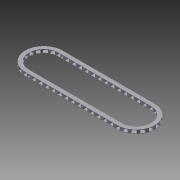
# Autodesk Inventor part: chain
Saved by Autodesk Inventor 2011 (Build 150239000, 239)
## iProperties
Created: 2010-04-19
Part Number: chain
Document SubType Name: Modeling
Designer: lucio
Density: 2.71 g/cm^3
Material: Aluminum-6061
Author: lucio
Autodesk Inventor part; units mm, degrees
ref_plane "YZ Plane" through (0, 0, 0) normal (1, 0, 0) x (0, 1, 0)
ref_plane "XZ Plane" through (0, 0, 0) normal (0, 1, 0) x (-1, 0, 0)
ref_plane "XY Plane" through (0, 0, 0) normal (0, 0, 1) x (1, 0, 0)
sketch "Sketch1" plane through (0, 0, 0) normal (0, 0, 1) x (1, 0, 0)
  line L0 (25, 0) -> (150, 0)
  line L1 (175, 25) -> (175, 25)
  line L2 (150, 50) -> (25, 50)
  line L3 (0, 25) -> (0, 25)
  arc A0 (25, 50) -> (0, 25) centre (25, 25) ccw
  arc A1 (175, 25) -> (150, 50) centre (150, 25) ccw
  arc A2 (150, 0) -> (175, 25) centre (150, 25) ccw
  arc A3 (0, 25) -> (25, 0) centre (25, 25) ccw
  line L4 (25, 45) -> (150, 45)
  line L5 (170, 25) -> (170, 25)
  line L6 (150, 5) -> (25, 5)
  line L7 (5, 25) -> (5, 25)
  arc A4 (25, 45) -> (5, 25) centre (25, 25) ccw
  arc A5 (5, 25) -> (25, 5) centre (25, 25) ccw
  arc A6 (150, 5) -> (170, 25) centre (150, 25) ccw
  arc A7 (170, 25) -> (150, 45) centre (150, 25) ccw
  line L8 (22.5, 25) -> (27.5, 25)
  line L9 (27.5, 25) -> (27.5, 50)
  line L10 (27.5, 50) -> (22.5, 50)
  line L11 (22.5, 50) -> (22.5, 25)
  line L12 (22.6508, 24.1449) -> (27.3492, 25.8551)
  line L13 (27.3492, 25.8551) -> (18.7987, 49.3474)
  line L14 (18.7987, 49.3474) -> (14.1003, 47.6373)
  line L15 (14.1003, 47.6373) -> (22.6508, 24.1449)
  line L16 (23.0849, 23.393) -> (26.9151, 26.607)
  line L17 (26.9151, 26.607) -> (10.8454, 45.7581)
  line L18 (10.8454, 45.7581) -> (7.0152, 42.5441)
  line L19 (7.0152, 42.5441) -> (23.0849, 23.393)
  line L20 (23.75, 22.8349) -> (26.25, 27.1651)
  line L21 (26.25, 27.1651) -> (4.5994, 39.6651)
  line L22 (4.5994, 39.6651) -> (2.0994, 35.3349)
  line L23 (2.0994, 35.3349) -> (23.75, 22.8349)
  line L24 (24.5659, 22.538) -> (25.4341, 27.462)
  line L25 (25.4341, 27.462) -> (0.8139, 31.8032)
  line L26 (0.8139, 31.8032) -> (-0.0543, 26.8792)
  line L27 (-0.0543, 26.8792) -> (24.5659, 22.538)
  line L28 (25.4341, 22.538) -> (24.5659, 27.462)
  line L29 (24.5659, 27.462) -> (-0.0543, 23.1208)
  line L30 (-0.0543, 23.1208) -> (0.8139, 18.1968)
  line L31 (0.8139, 18.1968) -> (25.4341, 22.538)
  line L32 (26.25, 22.8349) -> (23.75, 27.1651)
  line L33 (23.75, 27.1651) -> (2.0994, 14.6651)
  line L34 (2.0994, 14.6651) -> (4.5994, 10.3349)
  line L35 (4.5994, 10.3349) -> (26.25, 22.8349)
  line L36 (26.9151, 23.393) -> (23.0849, 26.607)
  line L37 (23.0849, 26.607) -> (7.0152, 7.4559)
  line L38 (7.0152, 7.4559) -> (10.8454, 4.2419)
  line L39 (10.8454, 4.2419) -> (26.9151, 23.393)
  line L40 (27.3492, 24.1449) -> (22.6508, 25.8551)
  line L41 (22.6508, 25.8551) -> (14.1003, 2.3627)
  line L42 (14.1003, 2.3627) -> (18.7987, 0.6526)
  line L43 (18.7987, 0.6526) -> (27.3492, 24.1449)
  line L44 (27.5, 25) -> (22.5, 25)
  line L45 (22.5, 25) -> (22.5, 0)
  line L46 (22.5, 0) -> (27.5, 0)
  line L47 (27.5, 0) -> (27.5, 25)
  line L48 (147.5, 24.9667) -> (152.5, 24.9667)
  line L49 (152.5, 24.9667) -> (152.5, 51.0386)
  line L50 (152.0822, 51.0326) -> (147.5, 50.9667)
  line L51 (147.5, 50.9667) -> (147.5, 24.9667)
  line L52 (147.6394, 25.8238) -> (152.3379, 24.1137)
  line L53 (152.3379, 24.1137) -> (161.255, 48.6133)
  line L54 (161.255, 48.6133) -> (156.5319, 50.2558)
  line L55 (156.5319, 50.2558) -> (147.6394, 25.8238)
  line L56 (148.0635, 26.5815) -> (151.8937, 23.3676)
  line L57 (151.8937, 23.3676) -> (168.6524, 43.3398)
  line L58 (168.6524, 43.3398) -> (164.776, 46.4986)
  line L59 (164.776, 46.4986) -> (148.0635, 26.5815)
  line L60 (148.7212, 27.1484) -> (151.2212, 22.8183)
  line L61 (151.2212, 22.8183) -> (173.8001, 35.8543)
  line L62 (173.8001, 35.8543) -> (171.2379, 40.1484)
  line L63 (171.2379, 40.1484) -> (148.7212, 27.1484)
  line L64 (149.5331, 27.4562) -> (150.4014, 22.5322)
  line L65 (150.4014, 22.5322) -> (176.0772, 27.0595)
  line L66 (176.0772, 27.0595) -> (175.1381, 31.9711)
  line L67 (175.1381, 31.9711) -> (149.5331, 27.4562)
  line L68 (150.4014, 27.4678) -> (149.5331, 22.5438)
  line L69 (149.5331, 22.5438) -> (175.2089, 18.0164)
  line L70 (175.2089, 18.0164) -> (176.0064, 22.9529)
  line L71 (176.0064, 22.9529) -> (150.4014, 27.4678)
  line L72 (151.2212, 27.1817) -> (148.7212, 22.8516)
  line L73 (148.7212, 22.8516) -> (171.3001, 9.8156)
  line L74 (171.3001, 9.8156) -> (173.7379, 14.1817)
  line L75 (173.7379, 14.1817) -> (151.2212, 27.1817)
  line L76 (151.8937, 26.6324) -> (148.0635, 23.4185)
  line L77 (148.0635, 23.4185) -> (164.8222, 3.4463)
  line L78 (164.8222, 3.4463) -> (168.6062, 6.7153)
  line L79 (168.6062, 6.7153) -> (151.8937, 26.6324)
  line L80 (152.3379, 25.8863) -> (147.6394, 24.1762)
  line L81 (147.6394, 24.1762) -> (156.5565, -0.3234)
  line L82 (156.5565, -0.3234) -> (161.2304, 1.4543)
  line L83 (161.2304, 1.4543) -> (152.3379, 25.8863)
  line L84 (152.5, 25.0333) -> (147.5, 25.0333)
  line L85 (147.5, 25.0333) -> (147.5, -1.0386)
  line L86 (147.5, -1.0386) -> (152.5, -0.9667)
  line L87 (152.5, -0.9667) -> (152.5, 25.0333)
  line L88 (143.785, 50) -> (138.785, 50)
  line L89 (138.785, 50) -> (138.785, -0.7152)
  line L90 (138.785, -0.7152) -> (143.785, -0.7152)
  line L91 (143.785, -0.7152) -> (143.785, 50)
  line L92 (135.07, 50) -> (130.07, 50)
  line L93 (130.07, 50) -> (130.07, 0)
  line L94 (130.07, 0) -> (135.07, 0)
  line L95 (135.07, 0) -> (135.07, 50)
  line L96 (126.355, 0) -> (121.355, 0)
  line L97 (121.355, 0) -> (121.355, 50)
  line L98 (121.355, 50) -> (126.355, 50)
  line L99 (126.355, 50) -> (126.355, 0)
  line L100 (117.64, 50) -> (112.64, 50)
  line L101 (112.64, 50) -> (112.64, 0)
  line L102 (112.64, 0) -> (117.64, 0)
  line L103 (117.64, 0) -> (117.64, 50)
  line L104 (108.925, 50) -> (103.925, 50)
  line L105 (103.925, 50) -> (103.925, 0)
  line L106 (103.925, 0) -> (108.925, 0)
  line L107 (108.925, 0) -> (108.925, 50)
  line L108 (100.21, 50) -> (95.21, 50)
  line L109 (95.21, 50) -> (95.21, 0)
  line L110 (95.21, 0) -> (100.21, 0)
  line L111 (100.21, 0) -> (100.21, 50)
  line L112 (91.495, 50) -> (86.495, 50)
  line L113 (86.495, 50) -> (86.495, 0)
  line L114 (86.495, 0) -> (91.495, 0)
  line L115 (91.495, 0) -> (91.495, 50)
  line L116 (82.78, 50) -> (77.78, 50)
  line L117 (77.78, 50) -> (77.78, 0)
  line L118 (77.78, 0) -> (82.78, 0)
  line L119 (82.78, 0) -> (82.78, 50)
  line L120 (74.065, 50) -> (69.065, 50)
  line L121 (69.065, 50) -> (69.065, 0)
  line L122 (69.065, 0) -> (74.065, 0)
  line L123 (74.065, 0) -> (74.065, 50)
  line L124 (65.35, 50) -> (60.35, 50)
  line L125 (60.35, 50) -> (60.35, 0)
  line L126 (60.35, 0) -> (65.35, 0)
  line L127 (65.35, 0) -> (65.35, 50)
  line L128 (56.635, 50) -> (51.635, 50)
  line L129 (51.635, 50) -> (51.635, 0)
  line L130 (51.635, 0) -> (56.635, 0)
  line L131 (56.635, 0) -> (56.635, 50)
  line L132 (47.92, 50) -> (42.92, 50)
  line L133 (42.92, 50) -> (42.92, 0)
  line L134 (42.92, 0) -> (47.92, 0)
  line L135 (47.92, 0) -> (47.92, 50)
  line L136 (39.205, 50) -> (34.205, 50)
  line L137 (34.205, 50) -> (34.205, 0)
  line L138 (34.205, 0) -> (39.205, 0)
  line L139 (39.205, 0) -> (39.205, 50)
  line L140 (30.49, 50) -> (27.6882, 50)
  line L141 (27.6882, 50) -> (27.6882, 0)
  line L142 (27.6882, 0) -> (30.49, 0)
  line L143 (30.49, 0) -> (30.49, 50)
  line L144 (152.0822, 51.0326) -> (147.5, 51.0326)
  line L145 (147.5, 51.0326) -> (147.5, 25.0333)
  line L146 (147.5, 25.0333) -> (152.0822, 25.0333)
  line L147 (152.0822, 25.0333) -> (152.0822, 51.0326)
  point P0 (0, 0)
  point P1 (175, 50)
  point P2 (175, 0)
  point P3 (0, 50)
  point P4 (170, 5)
  point P5 (170, 45)
  point P6 (5, 5)
  point P7 (16.4495, 48.4923)
  point P8 (18.1596, 43.7939)
  point P9 (8.9303, 44.1511)
  point P10 (12.1442, 40.3209)
  point P11 (3.3494, 37.5)
  point P12 (7.6795, 35)
  point P13 (0.3798, 29.3412)
  point P14 (5.3038, 28.473)
  point P15 (0.3798, 20.6588)
  point P16 (5.3038, 21.527)
  point P17 (3.3494, 12.5)
  point P18 (7.6795, 15)
  point P19 (8.9303, 5.8489)
  point P20 (12.1442, 9.6791)
  point P21 (16.4495, 1.5077)
  point P22 (18.1596, 6.2061)
  point P23 (25, 0)
  point P24 (25, 5)
  point P25 (158.5505, 48.4923)
  point P26 (156.8404, 43.7939)
  point P27 (166.0697, 44.1511)
  point P28 (162.8558, 40.3209)
  point P29 (171.6506, 37.5)
  point P30 (167.3205, 35)
  point P31 (174.6202, 29.3412)
  point P32 (169.6962, 28.473)
  point P33 (174.6202, 20.6588)
  point P34 (169.6962, 21.527)
  point P35 (171.6506, 12.5)
  point P36 (167.3205, 15)
  point P37 (166.0697, 5.8489)
  point P38 (162.8558, 9.6791)
  point P39 (158.5505, 1.5077)
  point P40 (156.8404, 6.2061)
  point P41 (150, 5)
  dimension "d0" = 175
  dimension "d1" = 50
  dimension "d2" = 25
  dimension "d3" = 165
  dimension "d4" = 40
  dimension "d6" = 20
  dimension "d11" = 2.5
  dimension "d12" = 5
  dimension "d15" = 180
  dimension "d19" = 2.5
  dimension "d20" = 5
  dimension "d23" = 180
  dimension "d27" = 5
  dimension "d28" = 3.715
  dimension "d29" = 3.715
  dimension "d30" = 3.715
  dimension "d31" = 5
  dimension "d32" = 5
  dimension "d33" = 3.715
  dimension "d34" = 5
  dimension "d35" = 3.715
  dimension "d36" = 5
  dimension "d37" = 3.715
  dimension "d38" = 5
  dimension "d39" = 3.715
  dimension "d40" = 5
  dimension "d41" = 3.715
  dimension "d42" = 5
  dimension "d43" = 3.715
  dimension "d44" = 5
  dimension "d45" = 3.715
  dimension "d46" = 5
  dimension "d47" = 3.715
  dimension "d48" = 5
  dimension "d49" = 3.715
  dimension "d50" = 5
  dimension "d51" = 3.715
  dimension "d52" = 5
  dimension "d53" = 2.8018
  dimension "d54" = 3.715
  dimension "d59" = 26
  dimension "d60" = 26
  constraints: 292 end point, 35 parallel, 18 horizontal, 18 perpendicular, 16 point on circle, 12 coincident, 12 tangent, 10 point on line, 8 centre point, 6 equal radius, 1 vertical, 294 other
  measures "d0" distance of point (0, 50) point (175, 50)
  measures "d1" distance of point (175, 50) point (175, 0)
  measures "d2" radius of A0
  measures "d3" distance of point (170, 5) point (5, 5)
  measures "d4" distance of point (170, 45) point (170, 5)
  measures "d6" radius of A4
  measures "d11" distance from line of A0.centre L11
  measures "d12" distance between parallel lines of L11 L9
  measures "d19" distance from line of L51 A1.centre
  measures "d20" distance between parallel lines of L49 L51
  measures "d27" distance between parallel lines of L91 L89
  measures "d28" distance between parallel lines of L51 L91
  measures "d29" distance between parallel lines of L99 L93
  measures "d30" distance between parallel lines of L95 L89
  measures "d31" distance between parallel lines of L93 L95
  measures "d32" distance between parallel lines of L97 L99
  measures "d33" distance between parallel lines of L103 L97
  measures "d34" distance between parallel lines of L101 L103
  measures "d35" distance between parallel lines of L107 L101
  measures "d36" distance between parallel lines of L105 L107
  measures "d37" distance between parallel lines of L111 L105
  measures "d38" distance between parallel lines of L109 L111
  measures "d39" distance between parallel lines of L109 L115
  measures "d40" distance between parallel lines of L113 L115
  measures "d41" distance between parallel lines of L119 L113
  measures "d42" distance between parallel lines of L117 L119
  measures "d43" distance between parallel lines of L123 L117
  measures "d44" distance between parallel lines of L121 L123
  measures "d45" distance between parallel lines of L127 L121
  measures "d46" distance between parallel lines of L125 L127
  measures "d47" distance between parallel lines of L131 L125
  measures "d48" distance between parallel lines of L129 L131
  measures "d49" distance between parallel lines of L135 L129
  measures "d50" distance between parallel lines of L133 L135
  measures "d51" distance between parallel lines of L133 L139
  measures "d52" distance between parallel lines of L137 L139
  measures "d53" distance between parallel lines of L141 L143
  measures "d54" distance between parallel lines of L143 L137
  measures "d59" distance of L50.end L48.start
  measures "d60" distance from line of A1.centre L50
extrude "Extrusion1" add sketch "Sketch1" along normal mid plane 5 contours A3 L45 A5 L6 L47 L0 | L47 L6 L141 L0 | A3 L43 A5 L45 | L141 L6 L143 L0 | A3 L41 A5 L43 | L143 L6 L137 L0 | L137 L6 L139 L0 | L141 L2 L143 L4 | L4 L9 L2 L141 | L4 A4 L11 A0 L2 L9 | A3 L39 A5 L41 | L139 L6 L133 L0 | L143 L2 L137 L4 | A3 L37 A5 L39 | L133 L6 L135 L0 | L137 L2 L139 L4 | A4 L13 A0 L11 | L37 A3 L35 A5 | L135 L6 L129 L0 | L139 L2 L133 L4 | A4 L15 A0 L13 | L35 A3 L33 A5 | L129 L6 L131 L0 | L133 L2 L135 L4 | A4 L17 A0 L15 | A4 L19 A0 L17 | L33 A3 L31 A5 | L131 L6 L125 L0 | L135 L2 L129 L4 | A4 L21 A0 L19 | A4 L23 A0 L21 | L31 A3 L29 A5 | L125 L6 L127 L0 | L129 L2 L131 L4 | A4 L25 A0 L23 | A4 L27 A0 L25 | L29 A3 A0 L27 A4 A5 | L127 L6 L121 L0 | L131 L2 L125 L4 | L121 L6 L123 L0 | L125 L2 L127 L4 | L123 L6 L117 L0 | L127 L2 L121 L4 | L117 L6 L119 L0 | L121 L2 L123 L4 | L119 L6 L113 L0 | L123 L2 L117 L4 | L113 L6 L115 L0 | L117 L2 L119 L4 | L115 L6 L109 L0 | L119 L2 L113 L4 | L109 L6 L111 L0 | L113 L2 L115 L4 | L111 L6 L105 L0 | L115 L2 L109 L4 | L105 L6 L107 L0 | L109 L2 L111 L4 | L107 L6 L101 L0 | L111 L2 L105 L4 | L101 L6 L103 L0 | L105 L2 L107 L4 | L103 L6 L97 L0 | L107 L2 L101 L4 | L97 L6 L99 L0 | L101 L2 L103 L4 | L99 L6 L93 L0 | L103 L2 L97 L4 | L93 L6 L95 L0 | L97 L2 L99 L4 | L95 L6 L89 L0 | L99 L2 L93 L4 | L89 L6 L91 L0 | L93 L2 L95 L4 | L91 L6 L85 L0 | L95 L2 L89 L4 | L85 L6 A6 L87 A2 L0 | L89 L2 L91 L4 | L91 L2 L51 L4 | L87 A6 L81 A2 | L51 L2 A1 L147 A7 L4 | L81 A6 L83 A2 | L83 A6 L77 A2 | L147 A1 L49 A7 | L77 A6 L79 A2 | L49 A1 L55 A7 | L79 A6 L73 A2 | L55 A1 L53 A7 | L73 A6 L75 A2 | L53 A1 L59 A7 | L75 A6 L69 A2 | L59 A1 L57 A7 | L69 A6 L71 A2 | L57 A1 L63 A7 | L71 A6 A7 L65 A1 A2 | L63 A1 L61 A7 | L61 A1 L67 A7 | L67 A1 L65 A7
extrude "Extrusion2" cut sketch "Sketch1" along normal mid plane 4 contours A3 L45 A5 L6 L47 L0 | L46 L45 A3 | L6 A5 L45 L43 L40 L8 L47 | L43 L42 A3 | A3 L41 A5 L43 | L8 L12 L13 L11 A4 L4 L9 | L42 L41 A3 | A5 L41 L39 L45 L43 | L45 L39 L36 L40 L43 | L12 L15 L45 L8 | L16 L19 L45 L15 L12 | L16 L17 L11 L13 L12 | L20 L23 L45 L19 L16 | L20 L21 L11 L17 L16 | L24 L27 L45 L23 L20 | L24 L25 L11 L21 L20 | L28 L31 L45 L27 L24 | L28 L29 L11 L25 L24 | L32 L35 L45 L31 L28 | L32 L33 L11 L29 L28 | L36 L39 L45 L35 L32 | L36 L37 L11 L33 L32 | L40 L41 L11 L37 L36 | L8 L11 L41 L40 | L4 A4 L11 A0 L2 L9 | L39 L41 L35 L45 | L45 L15 L41 L11 | L39 L38 A3 | A3 L37 A5 L39 | A5 L37 L35 L41 L39 | L35 L41 L31 L45 | L41 L15 L37 L11 | L45 L19 L41 L15 | L11 L17 L15 A4 L13 | L45 L23 L41 L19 | L11 L21 L15 L17 | L45 L27 L41 L23 | L11 L25 L15 L21 | L45 L31 L41 L27 | L11 L29 L15 L25 | L11 L33 L15 L29 | L11 L37 L15 L33 | A0 L11 L10 | L38 L37 A3 | L35 L37 L31 L41 | L41 L19 L37 L15 | A4 L15 A0 L13 | L41 L23 L37 L19 | L15 L21 L19 A4 L17 | L41 L27 L37 L23 | L15 L25 L19 L21 | L41 L31 L37 L27 | L15 L29 L19 L25 | L15 L33 L19 L29 | L15 L37 L19 L33 | L35 A3 L33 A5 | A5 L33 L31 L37 L35 | A0 L14 L13 | L37 L23 L33 L19 | A4 L19 A0 L17 | L37 L27 L33 L23 | L19 L25 L23 A4 L21 | L37 L31 L33 L27 | L19 L29 L23 L25 | L19 L33 L23 L29 | L35 L34 A3 | L15 L14 A0 | A0 L18 L17 | L33 L27 L29 L23 | A4 L23 A0 L21 | L33 L31 A5 L29 L27 | L23 L29 L27 A4 L25 | L34 L33 A3 | L31 A3 L29 A5 | L19 L18 A0 | A0 L22 L21 | A4 L27 A0 L25 | L31 L30 A3 | L23 L22 A0 | A0 L26 L25 | A3 L30 L29 | L27 L26 A0
extrude "Extrusion3" cut sketch "Sketch1" along normal mid plane 4 contours L85 L6 A6 L87 A2 L0 | L0 A2 L87 L86 L85 | L85 L48 L80 L81 L87 A6 L6 | L51 L84 L52 L48 | L51 L2 A1 L147 A7 L4 | L4 A7 L147 L55 L52 L84 L51 | L81 A6 L83 A2 | A2 L83 L82 L81 | L48 L76 L77 L87 L81 L80 | L51 L50 L147 A1 L2 | L81 L87 L77 L83 A6 | L84 L49 L48 | L48 L87 L53 L52 | L52 L55 L147 L59 L56 | L52 L53 L87 L57 L56 | L56 L59 L147 L63 L60 | L56 L57 L87 L61 L60 | L60 L63 L147 L67 L64 | L60 L61 L87 L65 L64 | L64 L67 L147 L71 L68 | L64 L65 L87 L69 L68 | L68 L71 L147 L75 L72 | L68 L69 L87 L73 L72 | L72 L75 L147 L79 L76 | L72 L73 L87 L77 L76 | L76 L79 L147 L80 | L80 L147 L84 | L145 L144 L50 | L77 A6 L79 A2 | A2 L79 L78 L77 | L87 L73 L83 L77 | L49 L83 L53 L87 | L147 L79 L49 L83 L80 | L80 L83 L49 L84 L147 | L55 L49 L59 L147 | L77 L83 L73 L79 A6 | L87 L69 L83 L73 | L53 L83 L57 L87 | L59 L49 L63 L147 | L57 L83 L61 L87 | L63 L49 L67 L147 | L61 L83 L65 L87 | L67 L49 L71 L147 | L65 L83 L69 L87 | L71 L49 L75 L147 | L75 L49 L79 L147 | L55 A1 L53 A7 | A7 L53 L59 L49 L55 | L73 A6 L75 A2 | A2 L75 L74 L73 | L83 L69 L79 L73 | L49 L79 L53 L83 | L53 L79 L57 L83 | L59 L53 L63 L49 | L57 L79 L61 L83 | L63 L53 L67 L49 | L61 L79 L65 L83 | L67 L53 L71 L49 | L65 L79 L69 L83 | L71 L53 L75 L49 | L75 L53 L79 L49 | L55 L54 L53 A1 | L73 L79 L69 L75 A6 | L53 L75 L57 L79 | L59 A7 L57 L63 L53 | L57 L75 L61 L79 | L63 L57 L67 L53 | L61 L75 L65 L79 | L67 L57 L71 L53 | L65 L75 L69 L79 | L71 L57 L75 L53 | L59 A1 L57 A7 | L69 A6 L71 A2 | A2 L71 L70 L69 | L57 L71 L61 L75 | L63 A7 L61 L67 L57 | L61 L71 L65 L75 | L67 L61 L71 L57 | L65 L71 A6 L69 L75 | L59 L58 L57 A1 | L63 A1 L61 A7 | L61 L67 A7 L65 L71 | L63 L62 L61 A1 | L67 A1 L65 A7 | A1 L67 L66 L65
extrude "Extrusion4" cut sketch "Sketch1" along normal mid plane 4 contours L141 L6 L143 L0 | L47 L9 L4 L141 L6 | L6 A5 L45 L43 L40 L8 L47 | A5 L43 L45 | L141 L4 L143 L6 | L8 L12 L13 L11 A4 L4 L9 | A5 L41 L39 L45 L43 | L45 L39 L36 L40 L43 | L137 L6 L139 L0 | L143 L4 L137 L6 | L141 L2 L143 L4 | L12 L15 L45 L8 | L16 L19 L45 L15 L12 | L16 L17 L11 L13 L12 | L20 L23 L45 L19 L16 | L20 L21 L11 L17 L16 | L24 L27 L45 L23 L20 | L24 L25 L11 L21 L20 | L28 L31 L45 L27 L24 | L28 L29 L11 L25 L24 | L32 L35 L45 L31 L28 | L32 L33 L11 L29 L28 | L36 L39 L45 L35 L32 | L36 L37 L11 L33 L32 | L40 L41 L11 L37 L36 | L8 L11 L41 L40 | A5 L39 L41 | L39 L41 L35 L45 | L137 L4 L139 L6 | L45 L15 L41 L11 | A5 L37 L35 L41 L39 | L35 L41 L31 L45 | L133 L6 L135 L0 | L139 L4 L133 L6 | L137 L2 L139 L4 | L41 L15 L37 L11 | L45 L19 L41 L15 | L13 A4 L11 | L11 L17 L15 A4 L13 | L45 L23 L41 L19 | L11 L21 L15 L17 | L45 L27 L41 L23 | L11 L25 L15 L21 | L45 L31 L41 L27 | L11 L29 L15 L25 | L11 L33 L15 L29 | L11 L37 L15 L33 | A5 L35 L37 | L35 L37 L31 L41 | L133 L4 L135 L6 | L41 L19 L37 L15 | L41 L23 L37 L19 | L17 A4 L15 | L15 L21 L19 A4 L17 | L41 L27 L37 L23 | L15 L25 L19 L21 | L41 L31 L37 L27 | L15 L29 L19 L25 | L15 L33 L19 L29 | L15 L37 L19 L33 | A5 L33 L31 L37 L35 | L129 L6 L131 L0 | L135 L4 L129 L6 | L133 L2 L135 L4 | L37 L23 L33 L19 | L37 L27 L33 L23 | L21 A4 L19 | L19 L25 L23 A4 L21 | L37 L31 L33 L27 | L19 L29 L23 L25 | L19 L33 L23 L29 | A5 L31 L33 | L129 L4 L131 L6 | L33 L27 L29 L23 | L33 L31 A5 L29 L27 | L25 A4 L23 | L23 L29 L27 A4 L25 | L125 L6 L127 L0 | L131 L4 L125 L6 | L129 L2 L131 L4 | L29 A5 A4 L27 | L125 L4 L127 L6 | L121 L6 L123 L0 | L127 L4 L121 L6 | L125 L2 L127 L4 | L121 L4 L123 L6 | L117 L6 L119 L0 | L123 L4 L117 L6 | L121 L2 L123 L4 | L117 L4 L119 L6 | L113 L6 L115 L0 | L119 L4 L113 L6 | L117 L2 L119 L4 | L113 L4 L115 L6 | L109 L6 L111 L0 | L115 L4 L109 L6 | L113 L2 L115 L4 | L109 L4 L111 L6 | L105 L6 L107 L0 | L111 L4 L105 L6 | L109 L2 L111 L4 | L105 L4 L107 L6 | L101 L6 L103 L0 | L107 L4 L101 L6 | L105 L2 L107 L4 | L101 L4 L103 L6 | L97 L6 L99 L0 | L103 L4 L97 L6 | L101 L2 L103 L4 | L97 L4 L99 L6 | L93 L6 L95 L0 | L99 L4 L93 L6 | L97 L2 L99 L4 | L93 L4 L95 L6 | L89 L6 L91 L0 | L0 L91 L90 L89 | L95 L4 L89 L6 | L93 L2 L95 L4 | L89 L4 L91 L6 | L91 L4 L51 L85 L6 | L89 L2 L91 L4 | L85 L48 L80 L81 L87 A6 L6 | L51 L84 L52 L48 | L4 A7 L147 L55 L52 L84 L51 | L87 L81 A6 | L48 L76 L77 L87 L81 L80 | L81 L87 L77 L83 A6 | L84 L49 L48 | L48 L87 L53 L52 | L52 L55 L147 L59 L56 | L52 L53 L87 L57 L56 | L56 L59 L147 L63 L60 | L56 L57 L87 L61 L60 | L60 L63 L147 L67 L64 | L60 L61 L87 L65 L64 | L64 L67 L147 L71 L68 | L64 L65 L87 L69 L68 | L68 L71 L147 L75 L72 | L68 L69 L87 L73 L72 | L72 L75 L147 L79 L76 | L72 L73 L87 L77 L76 | L76 L79 L147 L80 | L80 L147 L84 | A7 L49 L55 L147 | L83 L77 A6 | L87 L73 L83 L77 | L49 L83 L53 L87 | L147 L79 L49 L83 L80 | L80 L83 L49 L84 L147 | A7 L55 L49 | L55 L49 L59 L147 | L77 L83 L73 L79 A6 | L87 L69 L83 L73 | L53 L83 L57 L87 | L59 L49 L63 L147 | L57 L83 L61 L87 | L63 L49 L67 L147 | L61 L83 L65 L87 | L67 L49 L71 L147 | L65 L83 L69 L87 | L71 L49 L75 L147 | L75 L49 L79 L147 | A7 L53 L59 L49 L55 | L79 L73 A6 | L83 L69 L79 L73 | L49 L79 L53 L83 | L53 L79 L57 L83 | L59 L53 L63 L49 | L57 L79 L61 L83 | L63 L53 L67 L49 | L61 L79 L65 L83 | L67 L53 L71 L49 | L65 L79 L69 L83 | L71 L53 L75 L49 | L75 L53 L79 L49 | A7 L59 L53 | L73 L79 L69 L75 A6 | L53 L75 L57 L79 | L59 A7 L57 L63 L53 | L57 L75 L61 L79 | L63 L57 L67 L53 | L61 L75 L65 L79 | L67 L57 L71 L53 | L65 L75 L69 L79 | L71 L57 L75 L53 | L75 L69 A6 | L57 L71 L61 L75 | L63 A7 L61 L67 L57 | L57 A7 L63 | L61 L71 L65 L75 | L67 L61 L71 L57 | L65 L71 A6 L69 L75 | L61 L67 A7 L65 L71 | L61 A7 L67 | L65 A7 A6 L71
equation "\"d29\" = d28"
equation "\"d30\" = d28"
equation "\"d31\" = d27"
equation "\"d32\" = d20"
equation "\"d33\" = d28"
equation "\"d34\" = d27"
equation "\"d35\" = d28"
equation "\"d36\" = d20"
equation "\"d37\" = d28"
equation "\"d38\" = d20"
equation "\"d39\" = d28"
equation "\"d40\" = d20"
equation "\"d41\" = d28"
equation "\"d42\" = d20"
equation "\"d43\" = d28"
equation "\"d44\" = d20"
equation "\"d45\" = d28"
equation "\"d46\" = d20"
equation "\"d47\" = d28"
equation "\"d48\" = d20"
equation "\"d49\" = d28"
equation "\"d50\" = d20"
equation "\"d51\" = d28"
equation "\"d52\" = d20"
equation "\"d54\" = d28"
body "Solid1"
